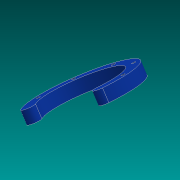
# Autodesk Inventor part: spacer
Saved by Autodesk Inventor 2020.3 (Build 243373000, 373)
## iProperties
Created: 2020-05-23
Part Number: spacer
Material: Generic
Document SubType Name: Modeling
Designer: Svend
Density: 1 g/cm^3
Appearance: Default
Author: Svend
Autodesk Inventor part; units mm, degrees
ref_plane "Work Plane1" through (-147.3677, -4.0754, 130.4495) normal (-0.5513437, 0.8342782, 0) x (0, 0, 1)
ref_plane "Work Plane2" through (-176.5966, 115.9868, 180.7146) normal (-0.5513437, 0.8342782, 0) x (0.1811695, 0.1197283, 0.9761366)
sketch "Sketch2" plane through (-176.5966, 115.9868, 180.7146) normal (-0.5513437, 0.8342782, 0) x (0.1811695, 0.1197283, 0.9761366)
  arc A0 (82.4936, -40) -> (107.4936, -33.3012) centre (82.4936, 10) ccw projected
  line L0 (107.4936, -33.3012) -> (126.4432, -22.3607) projected
  arc A1 (132.9687, -23.7251) -> (126.4432, -22.3607) centre (128.9432, -26.6908) ccw projected
  arc A2 (132.9687, -23.7251) -> (132.9687, 23.7251) centre (165.173, 0) ccw projected
  arc A3 (126.4432, 22.3607) -> (132.9687, 23.7251) centre (128.9432, 26.6908) ccw projected
  line L1 (126.4432, 22.3607) -> (107.4936, 33.3012) projected
  arc A4 (107.4936, 33.3012) -> (82.4936, 40) centre (82.4936, -10) ccw projected
  line L2 (-82.4936, 40) -> (82.4936, 40) projected
  arc A5 (-82.4936, 40) -> (-107.4936, 33.3012) centre (-82.4936, -10) ccw projected
  line L3 (-107.4936, 33.3012) -> (-126.4432, 22.3607) projected
  arc A6 (-132.9687, 23.7251) -> (-126.4432, 22.3607) centre (-128.9432, 26.6908) ccw projected
  arc A7 (-132.9687, 23.7251) -> (-132.9687, -23.7251) centre (-165.173, 0) ccw projected
  arc A8 (-126.4432, -22.3607) -> (-132.9687, -23.7251) centre (-128.9432, -26.6908) ccw projected
  line L4 (-126.4432, -22.3607) -> (-107.4936, -33.3012) projected
  arc A9 (-107.4936, -33.3012) -> (-82.4936, -40) centre (-82.4936, 10) ccw projected
  line L5 (82.4936, -40) -> (-82.4936, -40) projected
  arc A10 (3.6764, 4.0958) -> (3.6764, -4.0958) centre (6.5442, 0) ccw projected
  line L6 (3.6764, -4.0958) -> (20.5406, -15.9042) projected
  arc A11 (17.6727, -25) -> (20.5406, -15.9042) centre (17.6727, -20) ccw projected
  line L7 (17.6727, -25) -> (-19.8928, -25) projected
  arc A12 (-22.7607, -24.0958) -> (-19.8928, -25) centre (-19.8928, -20) ccw projected
  line L8 (-22.7607, -24.0958) -> (-51.3236, -4.0958) projected
  arc A13 (-51.3236, 4.0958) -> (-51.3236, -4.0958) centre (-48.4558, 0) ccw projected
  line L9 (-51.3236, 4.0958) -> (-22.7607, 24.0958) projected
  arc A14 (-19.8928, 25) -> (-22.7607, 24.0958) centre (-19.8928, 20) ccw projected
  line L10 (-19.8928, 25) -> (17.6727, 25) projected
  arc A15 (20.5406, 15.9042) -> (17.6727, 25) centre (17.6727, 20) ccw projected
  line L11 (20.5406, 15.9042) -> (3.6764, 4.0958) projected
  line L12 (-50.2924, 21.3617) -> (-62.1293, 13.0734) projected
  arc A16 (-64.2764, 12.9796) -> (-62.1293, 13.0734) centre (-63.2764, 14.7117) ccw projected
  line L13 (-64.2764, 12.9796) -> (-78.6322, 21.2679) projected
  arc A17 (-77.6322, 25) -> (-78.6322, 21.2679) centre (-77.6322, 23) ccw projected
  line L14 (-77.6322, 25) -> (-51.4395, 25) projected
  arc A18 (-50.2924, 21.3617) -> (-51.4395, 25) centre (-51.4395, 23) ccw projected
  line L15 (-62.1293, -13.0734) -> (-50.2924, -21.3617) projected
  arc A19 (-51.4395, -25) -> (-50.2924, -21.3617) centre (-51.4395, -23) ccw projected
  line L16 (-51.4395, -25) -> (-77.6322, -25) projected
  arc A20 (-78.6322, -21.2679) -> (-77.6322, -25) centre (-77.6322, -23) ccw projected
  line L17 (-78.6322, -21.2679) -> (-64.2764, -12.9796) projected
  arc A21 (-62.1293, -13.0734) -> (-64.2764, -12.9796) centre (-63.2764, -14.7117) ccw projected
  line L18 (-102.673, -23.5566) -> (-119.3236, -13.9434) projected
  arc A22 (-121.8236, -9.6132) -> (-119.3236, -13.9434) centre (-116.8236, -9.6132) ccw projected
  line L19 (-121.8236, -9.6132) -> (-121.8236, 9.6132) projected
  arc A23 (-119.3236, 13.9434) -> (-121.8236, 9.6132) centre (-116.8236, 9.6132) ccw projected
  line L20 (-119.3236, 13.9434) -> (-102.673, 23.5566) projected
  arc A24 (-97.673, 23.5566) -> (-102.673, 23.5566) centre (-100.173, 19.2265) ccw projected
  line L21 (-97.673, 23.5566) -> (-81.0224, 13.9434) projected
  arc A25 (-78.5224, 9.6132) -> (-81.0224, 13.9434) centre (-83.5224, 9.6132) ccw projected
  line L22 (-78.5224, 9.6132) -> (-78.5224, -9.6132) projected
  arc A26 (-81.0224, -13.9434) -> (-78.5224, -9.6132) centre (-83.5224, -9.6132) ccw projected
  line L23 (-81.0224, -13.9434) -> (-97.673, -23.5566) projected
  arc A27 (-102.673, -23.5566) -> (-97.673, -23.5566) centre (-100.173, -19.2265) ccw projected
  line L24 (72.827, -25) -> (57.1072, -25) projected
  arc A28 (54.2393, -24.0958) -> (57.1072, -25) centre (57.1072, -20) ccw projected
  line L25 (54.2393, -24.0958) -> (25.6764, -4.0958) projected
  arc A29 (25.6764, 4.0958) -> (25.6764, -4.0958) centre (28.5442, 0) ccw projected
  line L26 (25.6764, 4.0958) -> (54.2393, 24.0958) projected
  arc A30 (57.1072, 25) -> (54.2393, 24.0958) centre (57.1072, 20) ccw projected
  line L27 (57.1072, 25) -> (72.827, 25) projected
  arc A31 (77.827, 20) -> (72.827, 25) centre (72.827, 20) ccw projected
  line L28 (77.827, 20) -> (77.827, -20) projected
  arc A32 (72.827, -25) -> (77.827, -20) centre (72.827, -20) ccw projected
  circle A33 centre (-165.173, 0) radius 11 projected
  circle A34 centre (105.173, 0) radius 8 projected
  line L29 (87.4451, -10.7279) -> (97.4451, -10.7279) projected
  arc A35 (97.4451, -14.7279) -> (97.4451, -10.7279) centre (97.4451, -12.7279) ccw projected
  line L30 (97.4451, -14.7279) -> (87.4451, -14.7279) projected
  arc A36 (87.4451, -10.7279) -> (87.4451, -14.7279) centre (87.4451, -12.7279) ccw projected
  line L31 (122.9009, -14.7279) -> (112.9009, -14.7279) projected
  arc A37 (112.9009, -10.7279) -> (112.9009, -14.7279) centre (112.9009, -12.7279) ccw projected
  line L32 (112.9009, -10.7279) -> (122.9009, -10.7279) projected
  arc A38 (122.9009, -14.7279) -> (122.9009, -10.7279) centre (122.9009, -12.7279) ccw projected
  line L33 (97.4451, 10.7279) -> (87.4451, 10.7279) projected
  arc A39 (87.4451, 14.7279) -> (87.4451, 10.7279) centre (87.4451, 12.7279) ccw projected
  line L34 (87.4451, 14.7279) -> (97.4451, 14.7279) projected
  arc A40 (97.4451, 10.7279) -> (97.4451, 14.7279) centre (97.4451, 12.7279) ccw projected
  line L35 (122.9009, 10.7279) -> (112.9009, 10.7279) projected
  arc A41 (112.9009, 14.7279) -> (112.9009, 10.7279) centre (112.9009, 12.7279) ccw projected
  line L36 (112.9009, 14.7279) -> (122.9009, 14.7279) projected
  arc A42 (122.9009, 10.7279) -> (122.9009, 14.7279) centre (122.9009, 12.7279) ccw projected
  line L37 (169.046, 1) -> (169.973, 1) projected
  line L38 (169.973, 1) -> (169.973, -1) projected
  line L39 (169.973, -1) -> (169.046, -1) projected
  arc A43 (169.046, 1) -> (169.046, -1) centre (165.173, 0) ccw projected
  circle A44 centre (158.2448, -4) radius 2 projected
  circle A45 centre (172.1012, -4) radius 2 projected
  circle A46 centre (165.173, 8) radius 2 projected
  circle A47 centre (145.374, -19.799) radius 1.6 projected
  circle A48 centre (165.173, -28) radius 1.6 projected
  circle A49 centre (184.972, -19.799) radius 1.6 projected
  circle A50 centre (193.173, 0) radius 1.6 projected
  circle A51 centre (184.972, 19.799) radius 1.6 projected
  circle A52 centre (165.173, 28) radius 1.6 projected
  circle A53 centre (145.374, 19.799) radius 1.6 projected
  circle A54 centre (137.173, 0) radius 1.6 projected
  circle A55 centre (-165.173, -16.0004) radius 1.55 projected
  circle A56 centre (-149.1726, 0) radius 1.55 projected
  circle A57 centre (-165.173, 16.0004) radius 1.55 projected
  circle A58 centre (-181.1734, 0) radius 1.55 projected
  arc A59 (-141.0198, 17.7938) -> (-141.0198, -17.7938) centre (-165.173, 0) ccw
  arc A60 (-141.0198, 17.7938) -> (-121.4432, 13.7004) centre (-128.9432, 26.6908) ccw
  line L40 (-121.4432, 13.7004) -> (-102.4936, 24.641)
  arc A61 (-82.4936, 30) -> (-102.4936, 24.641) centre (-82.4936, -10) ccw
  line L41 (-82.4936, 30) -> (82.4936, 30)
  arc A62 (102.4936, 24.641) -> (82.4936, 30) centre (82.4936, -10) ccw
  line L42 (102.4936, 24.641) -> (121.4432, 13.7004)
  arc A63 (121.4432, 13.7004) -> (141.0198, 17.7938) centre (128.9432, 26.6908) ccw
  arc A64 (141.0198, -17.7938) -> (141.0198, 17.7938) centre (165.173, 0) ccw
  arc A65 (141.0198, -17.7938) -> (121.4432, -13.7004) centre (128.9432, -26.6908) ccw
  line L43 (121.4432, -13.7004) -> (102.4936, -24.641)
  arc A66 (82.4936, -30) -> (102.4936, -24.641) centre (82.4936, 10) ccw
  line L44 (82.4936, -30) -> (-82.4936, -30)
  arc A67 (-102.4936, -24.641) -> (-82.4936, -30) centre (-82.4936, 10) ccw
  line L45 (-102.4936, -24.641) -> (-121.4432, -13.7004)
  arc A68 (-121.4432, -13.7004) -> (-141.0198, -17.7938) centre (-128.9432, -26.6908) ccw
  arc A69 (-144.5699, -34.2857) -> (-149.7207, -25.7143) centre (-147.1453, -30) ccw
  line L46 (-205.173, 0) -> (-195.173, 0)
  arc A70 (-149.7207, 25.7143) -> (-144.5699, 34.2857) centre (-147.1453, 30) ccw
  point P0 (-158.2951, 120.6357)
  point P1 (-149.7207, 25.7143)
  point P2 (-144.5699, 34.2857)
  dimension "d4" = 10
  dimension "d5" = 30
  constraints: 28 point on circle, 14 end point, 12 centre point, 3 symmetric about line, 2 tangent, 16 other
  measures "d4" radial gap between concentric circles of A7 A59
  measures "d5" vertical distance of A33.centre A69.centre
extrude "Extrusion2" add sketch "Sketch2" along normal blind 10 contours A7 L46 A59 A69 | A7 A70 A59 L46
ref_plane "Work Plane3" through (-213.7676, 91.4218, -19.5622) normal (0.8143695, 0.5381868, -0.2171572) x (0.1811695, 0.1197283, 0.9761366)
sketch "Sketch3" plane through (-182.11, 124.3296, 180.7146) normal (-0.5513437, 0.8342782, 0) x (0.8143695, 0.5381868, -0.2171572)
  circle A0 centre (0, 200.673) radius 3.75 projected
  circle A1 centre (35.5, 165.173) radius 3.75 projected
  circle A2 centre (0, 129.673) radius 3.75 projected
  circle A3 centre (-35.5, 165.173) radius 3.75 projected
  circle A4 centre (-25.1023, 140.0707) radius 3.75 projected
  circle A5 centre (25.1023, 140.0707) radius 3.75 projected
  circle A6 centre (25.1023, 190.2753) radius 3.75 projected
  circle A7 centre (-25.1023, 190.2753) radius 3.75 projected
  circle A8 centre (0, 165.173) radius 40 projected
  circle A9 centre (0, 165.173) radius 30.089 projected
  point P0 (120.6357, 158.2951)
hole "Hole1" at (-218.4658, 100.3034, -15.1697) at (-196.1395, 115.058, -10.4712) at (-183.1242, 123.6594, 11.7741) at (-187.044, 121.0689, 38.5353) at (-205.6028, 108.8041, 54.136) at (-227.9291, 94.0495, 49.4376) at (-240.9444, 85.4481, 27.1923) at (-237.0246, 88.0386, 0.4311) direction (0.5513437, -0.8342782, 0) diameter 3 end through all
body "Solid2"
